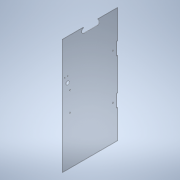
# Autodesk Inventor part: lc_box_side
Saved by Autodesk Inventor 2021.3 (Build 253353000, 353)
## iProperties
Created: 2019-07-19
Part Number: lc_box_side
Material: ポリカーボネート、クリア
Document SubType Name: Modeling
Designer: gisen
Density: 1.2 g/cm^3
Appearance: ポリカーボネート - クリア
Mass: 185.38 g
Surface Area: 1454.08 cm^2
Volume: 185.38 cm^3
Author: gisen
Autodesk Inventor part; units mm, degrees
ref_plane "YZ Plane" through (0, 0, 0) normal (1, 0, 0) x (0, 1, 0)
ref_plane "XZ Plane" through (0, 0, 0) normal (0, 1, 0) x (-1, 0, 0)
ref_plane "XY Plane" through (0, 0, 0) normal (0, 0, 1) x (1, 0, 0)
sketch "スケッチ1" plane through (0, 0, 0) normal (1, 0, 0) x (0, 1, 0)
  line L0 (125.6523, 179.1954) -> (-474.3477, 179.1954)
  line L1 (-474.3477, 179.1954) -> (-474.3477, -102.8046)
  line L2 (-474.3477, -102.8046) -> (125.6523, -102.8046)
  line L3 (125.6523, -102.8046) -> (125.6523, 179.1954)
  dimension "d0" = 600
  dimension "d1" = 282
  constraints: 8 end point, 2 parallel, 1 horizontal, 1 perpendicular
  measures "d0" distance of L0.start L0.end
  measures "d1" distance of L2.end L0.start
extrude "押し出し1" add sketch "スケッチ1" along normal blind 2.6
sketch "スケッチ4" plane through (2.6, 0, 0) normal (1, 0, 0) x (0, 0, -1)
  line L0 (102.8046, 125.6523) -> (-179.1954, 125.6523) projected
  line L1 (-179.1954, 125.6523) -> (-179.1954, -474.3477) projected
  point P0 (0, 0)
  point P1 (-139.1954, -225.3477)
  point P2 (-139.1954, -123.3477)
  dimension "d19" = 102
  dimension "d20" = 249
  dimension "d21" = 40
  dimension "d22" = 40
  measures "d19" distance of point (-139.195, -225.348) point (-139.195, -123.348)
  measures "d20" distance from line of point (-139.195, -123.348) L0
  measures "d21" distance from line of L1 point (-139.195, -123.348)
  measures "d22" distance from line of L1 point (-139.195, -225.348)
hole "穴2" at (2.6, -225.3477, 139.1954) at (2.6, -123.3477, 139.1954) direction (-1, 0, 0) diameter 6.6 end through all
sketch "スケッチ5" plane through (2.6, 0, 0) normal (1, 0, 0) x (0, 0, -1)
  line L0 (-179.1954, 125.6523) -> (-179.1954, -474.3477) projected
  line L1 (102.8046, 125.6523) -> (-179.1954, 125.6523) projected
  point P0 (-152.1954, -84.3477)
  dimension "d30" = 27
  dimension "d31" = 210
  measures "d30" distance from line of L0 point (-152.195, -84.348)
  measures "d31" distance from line of L1 point (-152.195, -84.348)
hole "穴3" at (2.6, -84.3477, 152.1954) direction (-1, 0, 0) diameter 18 end through all
sketch "スケッチ6" plane through (2.6, 0, 0) normal (1, 0, 0) x (0, 0, -1)
  line L0 (-179.1954, 125.6523) -> (-179.1954, -474.3477) projected
  circle A0 centre (-152.1954, -84.3477) radius 9 projected
  point P0 (0, 0)
  point P1 (-166.6954, -53.9477)
  point P2 (-151.6954, -53.9477)
  dimension "d39" = 12.5
  dimension "d40" = 27.5
  dimension "d41" = 30.4
  dimension "d42" = 30.4
  measures "d39" distance from line of L0 point (-166.695, -53.948)
  measures "d40" distance from line of L0 point (-151.695, -53.948)
  measures "d41" vertical distance of A0.centre point (-151.695, -53.948)
  measures "d42" vertical distance of A0.centre point (-166.695, -53.948)
hole "穴4" at (2.6, -53.9477, 166.6954) at (2.6, -53.9477, 151.6954) direction (-1, 0, 0) diameter 4.5 end through all
sketch "スケッチ7" plane through (2.6, 0, 0) normal (1, 0, 0) x (0, 0, -1)
  line L0 (102.8046, 125.6523) -> (-179.1954, 125.6523) projected
  line L1 (102.8046, -474.3477) -> (102.8046, 125.6523) projected
  line L2 (-179.1954, -474.3477) -> (102.8046, -474.3477) projected
  point P0 (0, 0)
  point P1 (84.0046, -56.9477)
  point P2 (84.0046, -291.9477)
  dimension "d50" = 182.6
  dimension "d51" = 18.8
  dimension "d52" = 18.8
  dimension "d53" = 182.4
  measures "d50" distance from line of L0 point (84.005, -56.948)
  measures "d51" distance from line of L1 point (84.005, -56.948)
  measures "d52" distance from line of L1 point (84.005, -291.948)
  measures "d53" distance from line of L2 point (84.005, -291.948)
hole "穴5" at (2.6, -56.9477, -84.0046) at (2.6, -291.9477, -84.0046) direction (-1, 0, 0) diameter 6.7 end through all
sketch "スケッチ8" plane through (2.6, 0, 0) normal (1, 0, 0) x (0, 0, -1)
  line L0 (102.8046, -474.3477) -> (102.8046, 125.6523) projected
  line L1 (102.8046, 125.6523) -> (107.8046, 125.6523)
  line L2 (117.7603, -23.9477) -> (102.8046, -23.9477)
  line L3 (102.8046, -89.9477) -> (117.7603, -89.9477)
  line L4 (107.8046, 125.6523) -> (107.8046, -474.3477)
  line L5 (107.8046, -474.3477) -> (102.8046, -474.3477)
  line L6 (102.8046, -258.9477) -> (107.8046, -258.9477)
  line L7 (102.8046, -324.9477) -> (107.8046, -324.9477)
  circle A0 centre (84.0046, -56.9477) radius 3.35 projected
  circle A1 centre (84.0046, -291.9477) radius 3.35 projected
  point P0 (0, 0)
  point P1 (107.8046, -23.9477)
  point P2 (107.8046, -89.9477)
  dimension "d61" = 5
  dimension "d62" = 33
  dimension "d63" = 33
  dimension "d64" = 33
  dimension "d65" = 33
  constraints: 14 end point, 6 point on line, 4 perpendicular, 2 parallel, 1 horizontal, 1 vertical
  measures "d61" distance of L0.end L1.end
  measures "d62" distance from line of L2 A0.centre
  measures "d63" distance from line of L3 A0.centre
  measures "d64" distance from line of L6 A1.centre
  measures "d65" distance from line of L7 A1.centre
extrude "押し出し3" add sketch "スケッチ8" against normal blind 2.6 contours L0 L7 L4 L5 | L0 L3 L4 L6 | L0 L1 L4 L2
sketch "スケッチ9" plane through (2.6, 0, 0) normal (1, 0, 0) x (0, 0, -1)
  ellipse E0 centre (-2.4593, 110.6523) end of major axis (-2.4593, 125.1521) minor radius 14.4996 (5.606, 98.6026) -> (5.606, 122.702) ccw
  line L0 (4.4935, 123.5363) -> (-99.9579, 123.5363) projected
  line L1 (-99.9579, 97.7683) -> (4.4935, 97.7683) projected
  ellipse E1 centre (-67.383, 110.6523) end of major axis (-67.383, 123.067) minor radius 12.4145 (-70.683, 122.6204) -> (-70.683, 98.6842) ccw projected
  line L2 (-70.683, 122.6204) -> (-70.683, 125.6523)
  line L3 (102.8046, 125.6523) -> (-179.1954, 125.6523) projected
  line L4 (5.7266, 122.6204) -> (5.7266, 125.6523)
  line L5 (5.7266, 125.6523) -> (-70.683, 125.6523)
  line L6 (6.1243, 98.9661) -> (4.4935, 97.7683)
  line L7 (-70.683, 98.6842) -> (-66.6998, 97.7683)
  point P0 (0, 0)
  constraints: 10 end point, 2 perpendicular, 2 point on line, 1 vertical, 8 other
extrude "押し出し4" cut sketch "スケッチ9" against normal blind 3
